Autodesk Fusion 360 part; units mm, degrees
note: some values were not read from the file. Chosen so that the rebuilt part matches the saved one: which bodies a step acts on. Set by a fixed rule: which sketch regions a step uses.
(part 4 of 5)
fillet "Fillet1'" radius 1 2 edges at (-68.425, -130.25, -19.5) (-53.825, -130.25, -19.5) on bodies 35 in component "edge-bracket_3d"
mirror "Mirror1" about plane through (0, 0, 0) normal (1, 0, 0) of bodies 35 makes body 36 in component "edge-bracket_3d"
pattern_circular "C-Pattern1''" count 4 over 360 about axis through (0, 0, 1.75) along (0, 0, 1) of bodies 35 36 makes body 37 at (139.5, -61.164856, -43.585564) makes body 38 at (61.164856, 139.5, -43.585564) makes body 39 at (-139.5, 61.164856, -43.585564) makes body 40 at (139.5, 61.164856, -43.585564) makes body 41 at (-61.164856, 139.5, -43.585564) makes body 42 at (-139.5, -61.164856, -43.585564) in component "edge-bracket_3d"
sketch "Sketch1 (4)" plane through (0, 139.5, 0) normal (0, 1, 0) x (-1, 0, 0) in component "sides"
  circle A0 centre (130.661165, -11.838835) radius 1.75
  circle A1 centre (130.661165, -37.161165) radius 1.75
  line L0 (122.236544, -3) -> (122.236544, -46)
  line L1 (122.236544, -46) -> (138.5, -46)
  line L2 (138.5, -46) -> (138.5, -3)
  line L3 (138.5, -3) -> (122.236544, -3)
  line L4 (142.5, -3) -> (-142.5, -3)
  line L5 (-142.5, -3) -> (-142.5, -46)
  line L6 (-142.5, -46) -> (142.5, -46)
  line L7 (142.5, -46) -> (142.5, -3)
  line L8 (139.5, -46) -> (139.5, -3)
  line L9 (142.5, -37.4) -> (139.5, -37.4)
  line L10 (142.5, -28.8) -> (139.5, -28.8)
  line L11 (142.5, -20.2) -> (139.5, -20.2)
  line L12 (142.5, -11.6) -> (139.5, -11.6)
  line L13 (142.5, -3) -> (139.5, -3)
  line L14 (0, -46) -> (0, -3) construction
  line L15 (-142.5, -37.4) -> (-139.5, -37.4)
  line L16 (-139.5, -46) -> (-139.5, -3)
  line L17 (-142.5, -28.8) -> (-139.5, -28.8)
  line L18 (-142.5, -20.2) -> (-139.5, -20.2)
  line L19 (-142.5, -11.6) -> (-139.5, -11.6)
  point P0 (143.5, -3)
  point P1 (139.5, -46)
  point P2 (-143.5, -3)
  point P3 (-139.5, -46)
  dimension "d354" = 3
  dimension "d355" = 3
  dimension "d356" = 8.6
  dimension "d357" = 43
  dimension "d360" = 0
  dimension "d361" = 34.4
  constraint horizontal L4
  constraint vertical L5
  constraint horizontal L6
  constraint vertical L7
  constraint coincident P3 L6
  constraint coincident P0 L4
  constraint coincident P1 L8.start
  constraint coincident L4 L8.end
  constraint perpendicular L4 L8
  constraint coincident L7 L9.start
  constraint coincident L8 L9.end
  constraint perpendicular L8 L9
  constraint midpoint L6 L14.start
  constraint midpoint L4 L14.end
  constraint symmetric P1 L14 P3
  constraint symmetric L8.end L14 L16.end
  constraint symmetric L9.start L14 L15.start
  constraint symmetric L9.end L14 L15.end
  constraint symmetric L10.start L14 L17.start
  constraint symmetric L10.end L14 L17.end
  constraint symmetric L11.start L14 L18.start
  constraint symmetric L11.end L14 L18.end
  constraint symmetric L12.start L14 L19.start
  constraint symmetric L12.end L14 L19.end
  measures "d354" distance of P1 L7
  measures "d355" distance of P3 L5
  measures "d356" distance of L6 L9
  measures "d357" distance of L4.start L6.end
extrude "Extrude1'''''" add sketch "Sketch1 (4)" along normal blind 3 separate body contours A0 | A1 | L0 L1 L2 L3 L4 L6 | L0 L4 L6 L16 | L2 L4 L6 L8 | L4 L7 L8 L12 L13 | L5 L16 L18 L19 | L6 L7 L8 L9 | L5 L15 L16 L17 | L7 L8 L10 L11 picked at (131.451099, -11.382766) picked at (129.871232, -36.705097) picked at (124.519186, -28.46729) picked at (34.991029, -23.066667) picked at (138.833333, -28.8) picked at (140.5, -8.733333) picked at (-141.5, -14.466667) picked at (140.5, -40.266667) picked at (-140.5, -34.533333) picked at (140.5, -23.066667) makes body 43 in component "sides"
sketch "Sketch2 (5)" plane through (0, 142.5, 0) normal (0, 1, 0) x (-1, 0, 0) in component "sides"
  line L0 (-142.5, -20.2) -> (-139.5, -20.2)
  line L1 (-139.5, -20.2) -> (-139.5, -28.8)
  line L2 (-139.5, -28.8) -> (-142.5, -28.8)
  line L3 (-142.5, -28.8) -> (-142.5, -37.4)
  line L4 (-142.5, -37.4) -> (-139.5, -37.4)
  line L5 (-139.5, -37.4) -> (-139.5, -46)
  line L6 (-139.5, -46) -> (142.5, -46)
  line L7 (142.5, -46) -> (142.5, -37.4)
  line L8 (142.5, -37.4) -> (139.5, -37.4)
  line L9 (139.5, -37.4) -> (139.5, -28.8)
  line L10 (139.5, -28.8) -> (142.5, -28.8)
  line L11 (142.5, -28.8) -> (142.5, -20.2)
  line L12 (142.5, -20.2) -> (139.5, -20.2)
  line L13 (139.5, -20.2) -> (139.5, -11.6)
  line L14 (139.5, -11.6) -> (142.5, -11.6)
  line L15 (142.5, -11.6) -> (142.5, -3)
  line L16 (142.5, -3) -> (-139.5, -3)
  line L17 (-139.5, -3) -> (-139.5, -11.6)
  line L18 (-139.5, -11.6) -> (-142.5, -11.6)
  line L19 (-142.5, -11.6) -> (-142.5, -20.2)
  circle A0 centre (130.661165, -11.838835) radius 1.75
  circle A1 centre (130.661165, -37.161165) radius 1.75
  line L20 (122.236544, -3) -> (122.236544, -46)
  line L21 (122.236544, -46) -> (138.5, -46)
  line L22 (138.5, -46) -> (138.5, -3)
  line L23 (138.5, -3) -> (122.236544, -3)
  line L24 (54.825, -3) -> (54.825, -46)
  line L25 (54.825, -46) -> (67.425, -46)
  line L26 (67.425, -46) -> (67.425, -3)
  line L27 (67.425, -3) -> (54.825, -3)
  circle A2 centre (61.125, -37.161165) radius 1.6
  circle A3 centre (61.125, -11.838835) radius 1.6
  line L28 (-54.825, -46) -> (-54.825, -3)
  line L29 (-54.825, -3) -> (-67.425, -3)
  line L30 (-67.425, -3) -> (-67.425, -46)
  line L31 (-67.425, -46) -> (-54.825, -46)
  circle A4 centre (-61.125, -37.161165) radius 1.6
  circle A5 centre (-61.125, -11.838835) radius 1.6
  circle A6 centre (-130.661165, -37.161165) radius 1.75
  circle A7 centre (-130.661165, -11.838835) radius 1.75
  line L32 (-122.236544, -46) -> (-122.236544, -3)
  line L33 (-122.236544, -3) -> (-138.5, -3)
  line L34 (-138.5, -3) -> (-138.5, -46)
  line L35 (-138.5, -46) -> (-122.236544, -46)
extrude "Extrude2'''" cut sketch "Sketch2 (5)" against normal blind 3 contours A0 | A1 | A2 | A3 | A4 | A5 | A6 | A7 picked at (131.451099, -11.382766) picked at (129.871232, -36.705097) picked at (61.391667, -36.38488) picked at (61.391667, -11.062549) picked at (-60.858333, -36.38488) picked at (-60.858333, -11.062549) picked at (-131.451099, -36.705097) picked at (-129.871232, -11.382766) bodies 43 in component "sides"
pattern_circular "C-Pattern1'''" count 4 over 360 about axis through (0, 0, 1.75) along (0, 0, 1) of bodies 43 makes body 44 at (-139.5, -19.873831, -28.537978) makes body 45 at (19.873831, -139.5, -28.537978) makes body 46 at (139.5, 19.873831, -28.537978) in component "sides"
sketch "Sketch3 (5)" plane through (0, 142.5, 0) normal (0, 1, 0) x (-1, 0, 0) in component "sides"
  circle A0 centre (-61.125, -11.838835) radius 1.6
  circle A1 centre (130.661165, -11.838835) radius 1.75
  circle A2 centre (61.125, -37.161165) radius 1.6
  circle A3 centre (-130.661165, -37.161165) radius 1.75
  circle A4 centre (-61.125, -37.161165) radius 1.6
  circle A5 centre (130.661165, -37.161165) radius 1.75
  circle A6 centre (61.125, -11.838835) radius 1.6
  circle A7 centre (-130.661165, -11.838835) radius 1.75
  line L0 (-142.5, -20.2) -> (-139.5, -20.2)
  line L1 (-139.5, -20.2) -> (-139.5, -28.8)
  line L2 (-139.5, -28.8) -> (-142.5, -28.8)
  line L3 (-142.5, -28.8) -> (-142.5, -37.4)
  line L4 (-142.5, -37.4) -> (-139.5, -37.4)
  line L5 (-139.5, -37.4) -> (-139.5, -46)
  line L6 (-139.5, -46) -> (142.5, -46)
  line L7 (142.5, -46) -> (142.5, -37.4)
  line L8 (142.5, -37.4) -> (139.5, -37.4)
  line L9 (139.5, -37.4) -> (139.5, -28.8)
  line L10 (139.5, -28.8) -> (142.5, -28.8)
  line L11 (142.5, -28.8) -> (142.5, -20.2)
  line L12 (142.5, -20.2) -> (139.5, -20.2)
  line L13 (139.5, -20.2) -> (139.5, -11.6)
  line L14 (139.5, -11.6) -> (142.5, -11.6)
  line L15 (142.5, -11.6) -> (142.5, -3)
  line L16 (142.5, -3) -> (-139.5, -3)
  line L17 (-139.5, -3) -> (-139.5, -11.6)
  line L18 (-139.5, -11.6) -> (-142.5, -11.6)
  line L19 (-142.5, -11.6) -> (-142.5, -20.2)
  line L20 (61.125, -37.161165) -> (-61.125, -11.838835) construction
  line L21 (0, -24.5) -> (0, -46) construction
  line L22 (122.25, -21) -> (-122.25, -21)
  circle A8 centre (0, -33.5) radius 5.5
  dimension "d368" = 11
  dimension "d369" = 25
  dimension "d370" = 12.5
  constraint midpoint L20 L21.start
  constraint coincident L6 L21.end
  constraint perpendicular L6 L21
  constraint coincident L21 A8.centre
  measures "d368" diameter of A8
  measures "d369" distance of L6 L22
  measures "d370" distance of L22 A8.centre
extrude "Extrude3''''" cut sketch "Sketch3 (5)" against normal blind 282 contours A8 picked at (0.137005, -35.084997) bodies 43 in component "sides"
sketch "Sketch3 (6)" plane through (0, 0, -18) normal (0, 0, -1) x (1, 0, 0) in component "bolt-holder_3d"
  arc A0 (-68.625, 128.75) -> (-69.625, 129.75) centre (-69.625, 128.75) ccw
  line L0 (-69.625, 129.75) -> (-116.02505, 129.75)
  arc A1 (-116.02505, 129.75) -> (-116.716711, 128.027778) centre (-116.02505, 128.75) ccw
  arc A2 (-115.999634, 117.256712) -> (-116.716711, 128.027778) centre (-122.25, 122.25) ccw
  arc A3 (-115.999634, 117.256712) -> (-115.925445, 115.925445) centre (-115.218338, 116.632551) ccw
  line L1 (-115.925445, 115.925445) -> (-101.292893, 101.292893)
  arc A4 (-101.292893, 101.292893) -> (-100.585786, 101) centre (-100.585786, 102) ccw
  line L2 (-100.585786, 101) -> (-99.5, 101)
  line L3 (-99.5, 101) -> (-99.5, 110.5)
  line L4 (-99.5, 110.5) -> (-87.5, 110.5)
  line L5 (-87.5, 110.5) -> (-87.5, 101)
  line L6 (-87.5, 101) -> (-87, 101)
  arc A5 (-87, 101) -> (-86, 102) centre (-87, 102) ccw
  line L7 (-86, 102) -> (-86, 108.5)
  line L8 (-86, 108.5) -> (-84, 108.5)
  line L9 (-84, 108.5) -> (-84, 102)
  arc A6 (-84, 102) -> (-83, 101) centre (-83, 102) ccw
  line L10 (-83, 101) -> (-82.5, 101)
  line L11 (-82.5, 101) -> (-82.5, 110.5)
  line L12 (-82.5, 110.5) -> (-70.5, 110.5)
  line L13 (-70.5, 110.5) -> (-70.5, 101)
  line L14 (-70.5, 101) -> (-70, 101)
  arc A7 (-70, 101) -> (-69, 102) centre (-70, 102) ccw
  line L15 (-69, 102) -> (-69, 108.5)
  line L16 (-69, 108.5) -> (-67, 108.5)
  line L17 (-67, 108.5) -> (-67, 102)
  arc A8 (-67, 102) -> (-66, 101) centre (-66, 102) ccw
  line L18 (-66, 101) -> (-65.5, 101)
  line L19 (-65.5, 101) -> (-65.5, 110.5)
  line L20 (-65.5, 110.5) -> (-53.5, 110.5)
  line L21 (-53.5, 110.5) -> (-53.5, 101)
  line L22 (-53.5, 101) -> (-53, 101)
  arc A9 (-53, 101) -> (-52, 102) centre (-53, 102) ccw
  line L23 (-52, 102) -> (-52, 108.5)
  line L24 (-52, 108.5) -> (-50, 108.5)
  line L25 (-50, 108.5) -> (-50, 102)
  arc A10 (-50, 102) -> (-49, 101) centre (-49, 102) ccw
  line L26 (-49, 101) -> (-48.5, 101)
  line L27 (-48.5, 101) -> (-48.5, 110.5)
  line L28 (-48.5, 110.5) -> (-36.5, 110.5)
  line L29 (-36.5, 110.5) -> (-36.5, 101)
  line L30 (-36.5, 101) -> (-36, 101)
  arc A11 (-36, 101) -> (-35, 102) centre (-36, 102) ccw
  line L31 (-35, 102) -> (-35, 108.5)
  line L32 (-35, 108.5) -> (-33, 108.5)
  line L33 (-33, 108.5) -> (-33, 102)
  arc A12 (-33, 102) -> (-32, 101) centre (-32, 102) ccw
  line L34 (-32, 101) -> (-31.5, 101)
  line L35 (-31.5, 101) -> (-31.5, 110.5)
  line L36 (-31.5, 110.5) -> (-19.5, 110.5)
  line L37 (-19.5, 110.5) -> (-19.5, 101)
  line L38 (-19.5, 101) -> (-19, 101)
  arc A13 (-19, 101) -> (-18, 102) centre (-19, 102) ccw
  line L39 (-18, 102) -> (-18, 108.5)
  line L40 (-18, 108.5) -> (-16, 108.5)
  line L41 (-16, 108.5) -> (-16, 102)
  arc A14 (-16, 102) -> (-15, 101) centre (-15, 102) ccw
  line L42 (-15, 101) -> (-14.5, 101)
  line L43 (-14.5, 101) -> (-14.5, 110.5)
  line L44 (-14.5, 110.5) -> (-2.5, 110.5)
  line L45 (-2.5, 110.5) -> (-2.5, 101)
  line L46 (-2.5, 101) -> (-2, 101)
  arc A15 (-2, 101) -> (-1, 102) centre (-2, 102) ccw
  line L47 (-1, 102) -> (-1, 108.5)
  line L48 (-1, 108.5) -> (1, 108.5)
  line L49 (1, 108.5) -> (1, 102)
  arc A16 (1, 102) -> (2, 101) centre (2, 102) ccw
  line L50 (2, 101) -> (2.5, 101)
  line L51 (2.5, 101) -> (2.5, 110.5)
  line L52 (2.5, 110.5) -> (14.5, 110.5)
  line L53 (14.5, 110.5) -> (14.5, 101)
  line L54 (14.5, 101) -> (15, 101)
  arc A17 (15, 101) -> (16, 102) centre (15, 102) ccw
  line L55 (16, 102) -> (16, 108.5)
  line L56 (16, 108.5) -> (18, 108.5)
  line L57 (18, 108.5) -> (18, 102)
  arc A18 (18, 102) -> (19, 101) centre (19, 102) ccw
  line L58 (19, 101) -> (19.5, 101)
  line L59 (19.5, 101) -> (19.5, 110.5)
  line L60 (19.5, 110.5) -> (31.5, 110.5)
  line L61 (31.5, 110.5) -> (31.5, 101)
  line L62 (31.5, 101) -> (32, 101)
  arc A19 (32, 101) -> (33, 102) centre (32, 102) ccw
  line L63 (33, 102) -> (33, 108.5)
  line L64 (33, 108.5) -> (35, 108.5)
  line L65 (35, 108.5) -> (35, 102)
  arc A20 (35, 102) -> (36, 101) centre (36, 102) ccw
  line L66 (36, 101) -> (36.5, 101)
  line L67 (36.5, 101) -> (36.5, 110.5)
  line L68 (36.5, 110.5) -> (48.5, 110.5)
  line L69 (48.5, 110.5) -> (48.5, 101)
  line L70 (48.5, 101) -> (49, 101)
  arc A21 (49, 101) -> (50, 102) centre (49, 102) ccw
  line L71 (50, 102) -> (50, 108.5)
  line L72 (50, 108.5) -> (52, 108.5)
  line L73 (52, 108.5) -> (52, 102)
  arc A22 (52, 102) -> (53, 101) centre (53, 102) ccw
  line L74 (53, 101) -> (53.5, 101)
  line L75 (53.5, 101) -> (53.5, 110.5)
  line L76 (53.5, 110.5) -> (65.5, 110.5)
  line L77 (65.5, 110.5) -> (65.5, 101)
  line L78 (65.5, 101) -> (66, 101)
  arc A23 (66, 101) -> (67, 102) centre (66, 102) ccw
  line L79 (67, 102) -> (67, 108.5)
  line L80 (67, 108.5) -> (69, 108.5)
  line L81 (69, 108.5) -> (69, 102)
  arc A24 (69, 102) -> (70, 101) centre (70, 102) ccw
  line L82 (70, 101) -> (70.5, 101)
  line L83 (70.5, 101) -> (70.5, 110.5)
  line L84 (70.5, 110.5) -> (82.5, 110.5)
  line L85 (82.5, 110.5) -> (82.5, 101)
  line L86 (82.5, 101) -> (83, 101)
  arc A25 (83, 101) -> (84, 102) centre (83, 102) ccw
  line L87 (84, 102) -> (84, 108.5)
  line L88 (84, 108.5) -> (86, 108.5)
  line L89 (86, 108.5) -> (86, 102)
  arc A26 (86, 102) -> (87, 101) centre (87, 102) ccw
  line L90 (87, 101) -> (87.5, 101)
  line L91 (87.5, 101) -> (87.5, 110.5)
  line L92 (87.5, 110.5) -> (99.5, 110.5)
  line L93 (99.5, 110.5) -> (99.5, 101)
  line L94 (99.5, 101) -> (100.585786, 101)
  arc A27 (100.585786, 101) -> (101.292893, 101.292893) centre (100.585786, 102) ccw
  line L95 (101.292893, 101.292893) -> (116.946699, 116.946699)
  arc A28 (116.946699, 116.946699) -> (122.25, 129.75) centre (122.25, 122.25) ccw
  line L96 (122.25, 129.75) -> (69.625, 129.75)
  arc A29 (69.625, 129.75) -> (68.625, 128.75) centre (69.625, 128.75) ccw
  line L97 (68.625, 128.75) -> (68.625, 122.25)
  arc A30 (53.625, 122.25) -> (68.625, 122.25) centre (61.125, 122.25) ccw
  line L98 (53.625, 122.25) -> (53.625, 128.75)
  arc A31 (53.625, 128.75) -> (52.625, 129.75) centre (52.625, 128.75) ccw
  line L99 (52.625, 129.75) -> (-52.625, 129.75)
  arc A32 (-52.625, 129.75) -> (-53.625, 128.75) centre (-52.625, 128.75) ccw
  line L100 (-53.625, 128.75) -> (-53.625, 122.25)
  arc A33 (-68.625, 122.25) -> (-53.625, 122.25) centre (-61.125, 122.25) ccw
  line L101 (-68.625, 122.25) -> (-68.625, 128.75)
  circle A34 centre (122.25, 122.25) radius 2.5
  line L102 (-12.5, 124.5) -> (-4.5, 124.5)
  arc A35 (4.5, 124.5) -> (-4.5, 124.5) centre (0, 118.5) ccw
  line L103 (4.5, 124.5) -> (12.5, 124.5)
  arc A36 (21.5, 124.5) -> (12.5, 124.5) centre (17, 118.5) ccw
  line L104 (21.5, 124.5) -> (29.5, 124.5)
  arc A37 (38.5, 124.5) -> (29.5, 124.5) centre (34, 118.5) ccw
  line L105 (38.5, 124.5) -> (51, 124.5)
  line L106 (51, 124.5) -> (51, 112.5)
  line L107 (51, 112.5) -> (38.5, 112.5)
  arc A38 (29.5, 112.5) -> (38.5, 112.5) centre (34, 118.5) ccw
  line L108 (29.5, 112.5) -> (21.5, 112.5)
  arc A39 (12.5, 112.5) -> (21.5, 112.5) centre (17, 118.5) ccw
  line L109 (12.5, 112.5) -> (4.5, 112.5)
  arc A40 (-4.5, 112.5) -> (4.5, 112.5) centre (0, 118.5) ccw
  line L110 (-4.5, 112.5) -> (-12.5, 112.5)
  arc A41 (-21.5, 112.5) -> (-12.5, 112.5) centre (-17, 118.5) ccw
  line L111 (-21.5, 112.5) -> (-29.5, 112.5)
  arc A42 (-38.5, 112.5) -> (-29.5, 112.5) centre (-34, 118.5) ccw
  line L112 (-38.5, 112.5) -> (-51, 112.5)
  line L113 (-51, 112.5) -> (-51, 124.5)
  line L114 (-51, 124.5) -> (-38.5, 124.5)
  arc A43 (-29.5, 124.5) -> (-38.5, 124.5) centre (-34, 118.5) ccw
  line L115 (-29.5, 124.5) -> (-21.5, 124.5)
  arc A44 (-12.5, 124.5) -> (-21.5, 124.5) centre (-17, 118.5) ccw
  arc A45 (-29.5, 112.5) -> (-29.5, 124.5) centre (-34, 118.5) ccw
  line L116 (-29.5, 112.5) -> (-21.5, 112.5)
  arc A46 (-21.5, 124.5) -> (-21.5, 112.5) centre (-17, 118.5) ccw
  line L117 (-21.5, 124.5) -> (-29.5, 124.5)
  line L118 (-51, 124.5) -> (-51, 112.5)
  line L119 (-51, 112.5) -> (-38.5, 112.5)
  arc A47 (-38.5, 124.5) -> (-38.5, 112.5) centre (-34, 118.5) ccw
  line L120 (-38.5, 124.5) -> (-51, 124.5)
  arc A48 (-12.5, 112.5) -> (-12.5, 124.5) centre (-17, 118.5) ccw
  line L121 (-12.5, 112.5) -> (-4.5, 112.5)
  arc A49 (-4.5, 124.5) -> (-4.5, 112.5) centre (0, 118.5) ccw
  line L122 (-4.5, 124.5) -> (-12.5, 124.5)
  arc A50 (4.5, 112.5) -> (4.5, 124.5) centre (0, 118.5) ccw
  line L123 (4.5, 112.5) -> (12.5, 112.5)
  arc A51 (12.5, 124.5) -> (12.5, 112.5) centre (17, 118.5) ccw
  line L124 (12.5, 124.5) -> (4.5, 124.5)
  arc A52 (21.5, 112.5) -> (21.5, 124.5) centre (17, 118.5) ccw
  line L125 (21.5, 112.5) -> (29.5, 112.5)
  arc A53 (29.5, 124.5) -> (29.5, 112.5) centre (34, 118.5) ccw
  line L126 (29.5, 124.5) -> (21.5, 124.5)
  line L127 (51, 124.5) -> (38.5, 124.5)
  arc A54 (38.5, 112.5) -> (38.5, 124.5) centre (34, 118.5) ccw
  line L128 (38.5, 112.5) -> (51, 112.5)
  line L129 (51, 112.5) -> (51, 124.5)
  line L130 (110.5, 70.5) -> (105.75, 70.5)
  line L131 (105.75, 70.5) -> (105.75, 82.5)
  line L132 (105.75, 82.5) -> (110.5, 82.5)
  line L133 (110.5, 82.5) -> (110.5, 70.5)
  circle A55 centre (122.25, 61.125) radius 1.6
  line L134 (110.5, 87.5) -> (105.75, 87.5)
  line L135 (105.75, 87.5) -> (105.75, 99.5)
  line L136 (105.75, 99.5) -> (110.5, 99.5)
  line L137 (110.5, 99.5) -> (110.5, 87.5)
  line L138 (51, -124.5) -> (46.25, -124.5)
  line L139 (46.25, -124.5) -> (46.25, -112.5)
  line L140 (46.25, -112.5) -> (51, -112.5)
  line L141 (51, -112.5) -> (51, -124.5)
  circle A56 centre (0, 118.5) radius 7.5
  circle A57 centre (-61.125, -122.25) radius 1.6
  circle A58 centre (61.125, -122.25) radius 1.6
  circle A59 centre (122.25, -61.125) radius 1.6
  circle A60 centre (-61.125, 122.25) radius 1.6
  circle A61 centre (61.125, 122.25) radius 1.6
  circle A62 centre (-122.25, -61.125) radius 1.6
  circle A63 centre (-122.25, 61.125) radius 1.6
  circle A64 centre (-34, 123) radius 1.6
  circle A65 centre (-17, 123) radius 1.6
  circle A66 centre (17, 123) radius 1.6
  circle A67 centre (34, 123) radius 1.6
  circle A68 centre (-34, 114) radius 1.6
  circle A69 centre (17, 114) radius 1.6
  circle A70 centre (-17, 114) radius 1.6
  circle A71 centre (34, 114) radius 1.6
  circle A72 centre (-122.25, 122.25) radius 2.5
  circle A73 centre (-122.25, -122.25) radius 2.5
  line L142 (-105.75, -2.5) -> (-105.75, -14.5)
  line L143 (-105.75, -14.5) -> (-110.5, -14.5)
  line L144 (-110.5, -14.5) -> (-110.5, -2.5)
  line L145 (-110.5, -2.5) -> (-105.75, -2.5)
  line L146 (-105.75, -87.5) -> (-105.75, -99.5)
  line L147 (-105.75, -99.5) -> (-110.5, -99.5)
  line L148 (-110.5, -99.5) -> (-110.5, -87.5)
  line L149 (-110.5, -87.5) -> (-105.75, -87.5)
  circle A74 centre (122.25, 122.25) radius 2.5
  line L150 (-105.75, -19.5) -> (-105.75, -31.5)
  line L151 (-105.75, -31.5) -> (-110.5, -31.5)
  line L152 (-110.5, -31.5) -> (-110.5, -19.5)
  line L153 (-110.5, -19.5) -> (-105.75, -19.5)
  line L154 (-105.75, -36.5) -> (-105.75, -48.5)
  line L155 (-105.75, -48.5) -> (-110.5, -48.5)
  line L156 (-110.5, -48.5) -> (-110.5, -36.5)
  line L157 (-110.5, -36.5) -> (-105.75, -36.5)
  line L158 (-105.75, -53.5) -> (-105.75, -65.5)
  line L159 (-105.75, -65.5) -> (-110.5, -65.5)
  line L160 (-110.5, -65.5) -> (-110.5, -53.5)
  line L161 (-110.5, -53.5) -> (-105.75, -53.5)
  line L162 (-105.75, -70.5) -> (-105.75, -82.5)
  line L163 (-105.75, -82.5) -> (-110.5, -82.5)
  line L164 (-110.5, -82.5) -> (-110.5, -70.5)
  line L165 (-110.5, -70.5) -> (-105.75, -70.5)
  line L166 (-46.25, -112.5) -> (-46.25, -124.5)
  line L167 (-46.25, -124.5) -> (-51, -124.5)
  line L168 (-51, -124.5) -> (-51, -112.5)
  line L169 (-51, -112.5) -> (-46.25, -112.5)
  line L170 (-105.75, 14.5) -> (-105.75, 2.5)
  line L171 (-105.75, 2.5) -> (-110.5, 2.5)
  line L172 (-110.5, 2.5) -> (-110.5, 14.5)
  line L173 (-110.5, 14.5) -> (-105.75, 14.5)
  line L174 (-105.75, 31.5) -> (-105.75, 19.5)
  line L175 (-105.75, 19.5) -> (-110.5, 19.5)
  line L176 (-110.5, 19.5) -> (-110.5, 31.5)
  line L177 (-110.5, 31.5) -> (-105.75, 31.5)
  line L178 (-105.75, 48.5) -> (-105.75, 36.5)
  line L179 (-105.75, 36.5) -> (-110.5, 36.5)
  line L180 (-110.5, 36.5) -> (-110.5, 48.5)
  line L181 (-110.5, 48.5) -> (-105.75, 48.5)
  line L182 (-105.75, 65.5) -> (-105.75, 53.5)
  line L183 (-105.75, 53.5) -> (-110.5, 53.5)
  line L184 (-110.5, 53.5) -> (-110.5, 65.5)
  line L185 (-110.5, 65.5) -> (-105.75, 65.5)
  line L186 (-105.75, 82.5) -> (-105.75, 70.5)
  line L187 (-105.75, 70.5) -> (-110.5, 70.5)
  line L188 (-110.5, 70.5) -> (-110.5, 82.5)
  line L189 (-110.5, 82.5) -> (-105.75, 82.5)
  line L190 (-105.75, 99.5) -> (-105.75, 87.5)
  line L191 (-105.75, 87.5) -> (-110.5, 87.5)
  line L192 (-110.5, 87.5) -> (-110.5, 99.5)
  line L193 (-110.5, 99.5) -> (-105.75, 99.5)
  line L194 (110.5, -99.5) -> (105.75, -99.5)
  line L195 (105.75, -99.5) -> (105.75, -87.5)
  line L196 (105.75, -87.5) -> (110.5, -87.5)
  line L197 (110.5, -87.5) -> (110.5, -99.5)
  line L198 (110.5, -82.5) -> (105.75, -82.5)
  line L199 (105.75, -82.5) -> (105.75, -70.5)
  line L200 (105.75, -70.5) -> (110.5, -70.5)
  line L201 (110.5, -70.5) -> (110.5, -82.5)
  line L202 (110.5, -65.5) -> (105.75, -65.5)
  line L203 (105.75, -65.5) -> (105.75, -53.5)
  line L204 (105.75, -53.5) -> (110.5, -53.5)
  line L205 (110.5, -53.5) -> (110.5, -65.5)
  line L206 (110.5, -48.5) -> (105.75, -48.5)
  line L207 (105.75, -48.5) -> (105.75, -36.5)
  line L208 (105.75, -36.5) -> (110.5, -36.5)
  line L209 (110.5, -36.5) -> (110.5, -48.5)
  line L210 (110.5, -31.5) -> (105.75, -31.5)
  line L211 (105.75, -31.5) -> (105.75, -19.5)
  line L212 (105.75, -19.5) -> (110.5, -19.5)
  line L213 (110.5, -19.5) -> (110.5, -31.5)
  line L214 (110.5, 36.5) -> (105.75, 36.5)
  line L215 (105.75, 36.5) -> (105.75, 48.5)
  line L216 (105.75, 48.5) -> (110.5, 48.5)
  line L217 (110.5, 48.5) -> (110.5, 36.5)
  line L218 (110.5, -14.5) -> (105.75, -14.5)
  line L219 (105.75, -14.5) -> (105.75, -2.5)
  line L220 (105.75, -2.5) -> (110.5, -2.5)
  line L221 (110.5, -2.5) -> (110.5, -14.5)
  line L222 (110.5, 53.5) -> (105.75, 53.5)
  line L223 (105.75, 53.5) -> (105.75, 65.5)
  line L224 (105.75, 65.5) -> (110.5, 65.5)
  line L225 (110.5, 65.5) -> (110.5, 53.5)
  line L226 (110.5, 2.5) -> (105.75, 2.5)
  line L227 (105.75, 2.5) -> (105.75, 14.5)
  line L228 (105.75, 14.5) -> (110.5, 14.5)
  line L229 (110.5, 14.5) -> (110.5, 2.5)
  line L230 (110.5, 19.5) -> (105.75, 19.5)
  line L231 (105.75, 19.5) -> (105.75, 31.5)
  line L232 (105.75, 31.5) -> (110.5, 31.5)
  line L233 (110.5, 31.5) -> (110.5, 19.5)
  circle A75 centre (122.25, -122.25) radius 2.5
  arc A76 (-129.75, -122.25) -> (-122.25, -129.75) centre (-122.25, -122.25) ccw
  line L234 (-122.25, -129.75) -> (122.25, -129.75)
  arc A77 (122.25, -129.75) -> (129.75, -122.25) centre (122.25, -122.25) ccw
  line L235 (129.75, -122.25) -> (129.75, 122.25)
  arc A78 (129.75, 122.25) -> (122.25, 129.75) centre (122.25, 122.25) ccw
  line L236 (122.25, 129.75) -> (-122.25, 129.75)
  arc A79 (-122.25, 129.75) -> (-129.75, 122.25) centre (-122.25, 122.25) ccw
  line L237 (-129.75, 122.25) -> (-129.75, -122.25)
  line L238 (-35.732051, 126) -> (-37.464102, 123)
  line L239 (-37.464102, 123) -> (-35.732051, 120)
  line L240 (-35.732051, 120) -> (-32.267949, 120)
  line L241 (-32.267949, 120) -> (-30.535898, 123)
  line L242 (-30.535898, 123) -> (-32.267949, 126)
  line L243 (-32.267949, 126) -> (-35.732051, 126)
  line L244 (-34, 118.5) -> (-17, 118.5) construction
  line L245 (-8.5, 124.5) -> (-8.5, 112.5)
  line L246 (-25.5, 124.5) -> (-25.5, 112.5) construction
  line L247 (-42.5, 124.5) -> (-42.5, 112.5)
  line L248 (-35.732051, 117) -> (-32.267949, 117)
  line L249 (-32.267949, 117) -> (-30.535898, 114)
  line L250 (-30.535898, 114) -> (-32.267949, 111)
  line L251 (-32.267949, 111) -> (-35.732051, 111)
  line L252 (-35.732051, 111) -> (-37.464102, 114)
  line L253 (-37.464102, 114) -> (-35.732051, 117)
  line L254 (-15.267949, 126) -> (-13.535898, 123)
  line L255 (-13.535898, 123) -> (-15.267949, 120)
  line L256 (-15.267949, 120) -> (-18.732051, 120)
  line L257 (-18.732051, 120) -> (-20.464102, 123)
  line L258 (-20.464102, 123) -> (-18.732051, 126)
  line L259 (-18.732051, 126) -> (-15.267949, 126)
  line L260 (-15.267949, 117) -> (-18.732051, 117)
  line L261 (-13.535898, 114) -> (-15.267949, 117)
  line L262 (-15.267949, 111) -> (-13.535898, 114)
  line L263 (-18.732051, 111) -> (-15.267949, 111)
  line L264 (-20.464102, 114) -> (-18.732051, 111)
  line L265 (-18.732051, 117) -> (-20.464102, 114)
  point P0 (-34, 123)
  dimension "d392" = 3
  constraint coincident P0 A64.centre
  constraint horizontal L240
  constraint coincident A42.centre A43.centre
  constraint coincident A41.centre A44.centre
  constraint midpoint L102 L245.start
  constraint midpoint L121 L245.end
  constraint midpoint L115 L246.start
  constraint midpoint L111 L246.end
  constraint symmetric L245.start L246 L247.start
  constraint symmetric L245.end L246 L247.end
  measures "d392" distance of P0 L243
extrude "Extrude2''''" add sketch "Sketch3 (6)" against normal blind 2.5 separate body contours A41 A44 A46 A48 L254 L255 L256 L257 L258 L260 L261 L262 L264 L265 | L102 L110 A48 L121 L122 L245 | L111 L115 A45 L116 A46 L117 | A42 A43 A45 A47 L238 L239 L240 L241 L242 L248 L249 L250 L252 L253 | L112 L114 L119 A47 L120 L247 picked at (-13.351657, 118.678175) picked at (-8.839691, 118.678175) picked at (-25.009344, 115.233041) picked at (-37.648343, 118.678175) picked at (-42.160309, 118.321825) makes body 47 in component "bolt-holder_3d"
sketch "Sketch4 (3)" plane through (0, 0, -15.5) normal (0, 0, 1) x (-1, 0, 0) in component "bolt-holder_3d"
  arc A0 (12.5, 112.5) -> (15.131402, 111.236506) centre (17, 118.5) ccw
  line L0 (15.131402, 111.236506) -> (13.535898, 114)
  line L1 (13.535898, 114) -> (15.267949, 117)
  line L2 (15.267949, 117) -> (18.732051, 117)
  line L3 (18.732051, 117) -> (20.464102, 114)
  line L4 (20.464102, 114) -> (18.868598, 111.236506)
  arc A1 (18.868598, 111.236506) -> (21.5, 112.5) centre (17, 118.5) ccw
  line L5 (21.5, 112.5) -> (29.5, 112.5)
  arc A2 (29.5, 112.5) -> (32.131402, 111.236506) centre (34, 118.5) ccw
  line L6 (32.131402, 111.236506) -> (30.535898, 114)
  line L7 (30.535898, 114) -> (32.267949, 117)
  line L8 (32.267949, 117) -> (35.732051, 117)
  line L9 (35.732051, 117) -> (37.464102, 114)
  line L10 (37.464102, 114) -> (35.868598, 111.236506)
  arc A3 (35.868598, 111.236506) -> (38.5, 112.5) centre (34, 118.5) ccw
  line L11 (38.5, 112.5) -> (42.5, 112.5)
  line L12 (42.5, 112.5) -> (42.5, 124.5)
  line L13 (42.5, 124.5) -> (38.5, 124.5)
  arc A4 (38.5, 124.5) -> (35.868598, 125.763494) centre (34, 118.5) ccw
  line L14 (35.868598, 125.763494) -> (37.464102, 123)
  line L15 (37.464102, 123) -> (35.732051, 120)
  line L16 (35.732051, 120) -> (32.267949, 120)
  line L17 (32.267949, 120) -> (30.535898, 123)
  line L18 (30.535898, 123) -> (32.131402, 125.763494)
  arc A5 (32.131402, 125.763494) -> (29.5, 124.5) centre (34, 118.5) ccw
  line L19 (29.5, 124.5) -> (21.5, 124.5)
  arc A6 (21.5, 124.5) -> (18.868598, 125.763494) centre (17, 118.5) ccw
  line L20 (18.868598, 125.763494) -> (20.464102, 123)
  line L21 (20.464102, 123) -> (18.732051, 120)
  line L22 (18.732051, 120) -> (15.267949, 120)
  line L23 (15.267949, 120) -> (13.535898, 123)
  line L24 (13.535898, 123) -> (15.131402, 125.763494)
  arc A7 (15.131402, 125.763494) -> (12.5, 124.5) centre (17, 118.5) ccw
  line L25 (12.5, 124.5) -> (8.5, 124.5)
  line L26 (8.5, 124.5) -> (8.5, 112.5)
  line L27 (8.5, 112.5) -> (12.5, 112.5)
  line L28 (-110.5, 70.5) -> (-105.75, 70.5)
  line L29 (-105.75, 70.5) -> (-105.75, 82.5)
  line L30 (-105.75, 82.5) -> (-110.5, 82.5)
  line L31 (-110.5, 82.5) -> (-110.5, 70.5)
  circle A8 centre (-122.25, 61.125) radius 1.6
  line L32 (-110.5, 87.5) -> (-105.75, 87.5)
  line L33 (-105.75, 87.5) -> (-105.75, 99.5)
  line L34 (-105.75, 99.5) -> (-110.5, 99.5)
  line L35 (-110.5, 99.5) -> (-110.5, 87.5)
  line L36 (-51, -124.5) -> (-46.25, -124.5)
  line L37 (-46.25, -124.5) -> (-46.25, -112.5)
  line L38 (-46.25, -112.5) -> (-51, -112.5)
  line L39 (-51, -112.5) -> (-51, -124.5)
  circle A9 centre (0, 118.5) radius 7.5
  circle A10 centre (61.125, -122.25) radius 1.6
  circle A11 centre (-61.125, -122.25) radius 1.6
  circle A12 centre (-122.25, -61.125) radius 1.6
  circle A13 centre (61.125, 122.25) radius 1.6
  circle A14 centre (-61.125, 122.25) radius 1.6
  circle A15 centre (122.25, -61.125) radius 1.6
  circle A16 centre (122.25, 61.125) radius 1.6
  circle A17 centre (34, 123) radius 1.6
  circle A18 centre (17, 123) radius 1.6
  circle A19 centre (-17, 123) radius 1.6
  circle A20 centre (-34, 123) radius 1.6
  circle A21 centre (34, 114) radius 1.6
  circle A22 centre (-17, 114) radius 1.6
  circle A23 centre (17, 114) radius 1.6
  circle A24 centre (-34, 114) radius 1.6
  circle A25 centre (122.25, 122.25) radius 2.5
  circle A26 centre (122.25, -122.25) radius 2.5
  line L40 (105.75, -2.5) -> (105.75, -14.5)
  line L41 (105.75, -14.5) -> (110.5, -14.5)
  line L42 (110.5, -14.5) -> (110.5, -2.5)
  line L43 (110.5, -2.5) -> (105.75, -2.5)
  line L44 (105.75, -87.5) -> (105.75, -99.5)
  line L45 (105.75, -99.5) -> (110.5, -99.5)
  line L46 (110.5, -99.5) -> (110.5, -87.5)
  line L47 (110.5, -87.5) -> (105.75, -87.5)
  circle A27 centre (-122.25, 122.25) radius 2.5
  line L48 (105.75, -19.5) -> (105.75, -31.5)
  line L49 (105.75, -31.5) -> (110.5, -31.5)
  line L50 (110.5, -31.5) -> (110.5, -19.5)
  line L51 (110.5, -19.5) -> (105.75, -19.5)
  line L52 (105.75, -36.5) -> (105.75, -48.5)
  line L53 (105.75, -48.5) -> (110.5, -48.5)
  line L54 (110.5, -48.5) -> (110.5, -36.5)
  line L55 (110.5, -36.5) -> (105.75, -36.5)
  line L56 (105.75, -53.5) -> (105.75, -65.5)
  line L57 (105.75, -65.5) -> (110.5, -65.5)
  line L58 (110.5, -65.5) -> (110.5, -53.5)
  line L59 (110.5, -53.5) -> (105.75, -53.5)
  line L60 (105.75, -70.5) -> (105.75, -82.5)
  line L61 (105.75, -82.5) -> (110.5, -82.5)
  line L62 (110.5, -82.5) -> (110.5, -70.5)
  line L63 (110.5, -70.5) -> (105.75, -70.5)
  line L64 (46.25, -112.5) -> (46.25, -124.5)
  line L65 (46.25, -124.5) -> (51, -124.5)
  line L66 (51, -124.5) -> (51, -112.5)
  line L67 (51, -112.5) -> (46.25, -112.5)
  line L68 (105.75, 14.5) -> (105.75, 2.5)
  line L69 (105.75, 2.5) -> (110.5, 2.5)
  line L70 (110.5, 2.5) -> (110.5, 14.5)
  line L71 (110.5, 14.5) -> (105.75, 14.5)
  line L72 (105.75, 31.5) -> (105.75, 19.5)
  line L73 (105.75, 19.5) -> (110.5, 19.5)
  line L74 (110.5, 19.5) -> (110.5, 31.5)
  line L75 (110.5, 31.5) -> (105.75, 31.5)
  line L76 (105.75, 48.5) -> (105.75, 36.5)
  line L77 (105.75, 36.5) -> (110.5, 36.5)
  line L78 (110.5, 36.5) -> (110.5, 48.5)
  line L79 (110.5, 48.5) -> (105.75, 48.5)
  line L80 (105.75, 65.5) -> (105.75, 53.5)
  line L81 (105.75, 53.5) -> (110.5, 53.5)
  line L82 (110.5, 53.5) -> (110.5, 65.5)
  line L83 (110.5, 65.5) -> (105.75, 65.5)
  line L84 (105.75, 82.5) -> (105.75, 70.5)
  line L85 (105.75, 70.5) -> (110.5, 70.5)
  line L86 (110.5, 70.5) -> (110.5, 82.5)
  line L87 (110.5, 82.5) -> (105.75, 82.5)
  line L88 (105.75, 99.5) -> (105.75, 87.5)
  line L89 (105.75, 87.5) -> (110.5, 87.5)
  line L90 (110.5, 87.5) -> (110.5, 99.5)
  line L91 (110.5, 99.5) -> (105.75, 99.5)
  line L92 (-110.5, -99.5) -> (-105.75, -99.5)
  line L93 (-105.75, -99.5) -> (-105.75, -87.5)
  line L94 (-105.75, -87.5) -> (-110.5, -87.5)
  line L95 (-110.5, -87.5) -> (-110.5, -99.5)
  line L96 (-110.5, -82.5) -> (-105.75, -82.5)
  line L97 (-105.75, -82.5) -> (-105.75, -70.5)
  line L98 (-105.75, -70.5) -> (-110.5, -70.5)
  line L99 (-110.5, -70.5) -> (-110.5, -82.5)
  line L100 (-110.5, -65.5) -> (-105.75, -65.5)
  line L101 (-105.75, -65.5) -> (-105.75, -53.5)
  line L102 (-105.75, -53.5) -> (-110.5, -53.5)
  line L103 (-110.5, -53.5) -> (-110.5, -65.5)
  line L104 (-110.5, -48.5) -> (-105.75, -48.5)
  line L105 (-105.75, -48.5) -> (-105.75, -36.5)
  line L106 (-105.75, -36.5) -> (-110.5, -36.5)
  line L107 (-110.5, -36.5) -> (-110.5, -48.5)
  line L108 (-110.5, -31.5) -> (-105.75, -31.5)
  line L109 (-105.75, -31.5) -> (-105.75, -19.5)
  line L110 (-105.75, -19.5) -> (-110.5, -19.5)
  line L111 (-110.5, -19.5) -> (-110.5, -31.5)
  line L112 (-110.5, 36.5) -> (-105.75, 36.5)
  line L113 (-105.75, 36.5) -> (-105.75, 48.5)
  line L114 (-105.75, 48.5) -> (-110.5, 48.5)
  line L115 (-110.5, 48.5) -> (-110.5, 36.5)
  line L116 (-110.5, -14.5) -> (-105.75, -14.5)
  line L117 (-105.75, -14.5) -> (-105.75, -2.5)
  line L118 (-105.75, -2.5) -> (-110.5, -2.5)
  line L119 (-110.5, -2.5) -> (-110.5, -14.5)
  line L120 (-110.5, 53.5) -> (-105.75, 53.5)
  line L121 (-105.75, 53.5) -> (-105.75, 65.5)
  line L122 (-105.75, 65.5) -> (-110.5, 65.5)
  line L123 (-110.5, 65.5) -> (-110.5, 53.5)
  line L124 (-110.5, 2.5) -> (-105.75, 2.5)
  line L125 (-105.75, 2.5) -> (-105.75, 14.5)
  line L126 (-105.75, 14.5) -> (-110.5, 14.5)
  line L127 (-110.5, 14.5) -> (-110.5, 2.5)
  line L128 (-110.5, 19.5) -> (-105.75, 19.5)
  line L129 (-105.75, 19.5) -> (-105.75, 31.5)
  line L130 (-105.75, 31.5) -> (-110.5, 31.5)
  line L131 (-110.5, 31.5) -> (-110.5, 19.5)
  circle A28 centre (-122.25, -122.25) radius 2.5
  arc A29 (122.25, -129.75) -> (129.75, -122.25) centre (122.25, -122.25) ccw
  line L132 (122.25, -129.75) -> (-122.25, -129.75)
  arc A30 (-129.75, -122.25) -> (-122.25, -129.75) centre (-122.25, -122.25) ccw
  line L133 (-129.75, -122.25) -> (-129.75, 122.25)
  arc A31 (-122.25, 129.75) -> (-129.75, 122.25) centre (-122.25, 122.25) ccw
  line L134 (-122.25, 129.75) -> (122.25, 129.75)
  arc A32 (129.75, 122.25) -> (122.25, 129.75) centre (122.25, 122.25) ccw
  line L135 (129.75, 122.25) -> (129.75, -122.25)
  arc A33 (38.5, 124.5) -> (29.5, 124.5) centre (34, 118.5) ccw
  arc A34 (38.5, 112.5) -> (38.5, 124.5) centre (34, 118.5) ccw
  arc A35 (29.5, 112.5) -> (38.5, 112.5) centre (34, 118.5) ccw
  arc A36 (29.5, 124.5) -> (29.5, 112.5) centre (34, 118.5) ccw
  circle A37 centre (34, 118.5) radius 7.5
  arc A38 (21.5, 124.5) -> (12.5, 124.5) centre (17, 118.5) ccw
  arc A39 (21.5, 112.5) -> (21.5, 124.5) centre (17, 118.5) ccw
  arc A40 (12.5, 112.5) -> (21.5, 112.5) centre (17, 118.5) ccw
  arc A41 (12.5, 124.5) -> (12.5, 112.5) centre (17, 118.5) ccw
  circle A42 centre (17, 118.5) radius 7.5
extrude "Extrude3'''''" add sketch "Sketch4 (3)" along normal blind 0.5 contours A0 L0 L1 L2 L3 L4 A1 A6 L20 L21 L22 L23 L24 A7 A38 A39 A40 A41 A42 | L25 L26 L27 A41 A42 | L0 L1 L2 L3 L4 A40 A42 | L20 L21 L22 L23 L24 A38 A42 | L5 L19 A36 A37 A39 A42 | A2 L6 L7 L8 L9 L10 A3 A4 L14 L15 L16 L17 L18 A5 A33 A34 A35 A36 A37 | L6 L7 L8 L9 L10 A35 A37 | L14 L15 L16 L17 L18 A33 A37 | L11 L12 L13 A34 A37 picked at (20.654701, 118.5) picked at (8.839691, 118.678175) picked at (14.787432, 115.231405) picked at (14.787432, 121.768595) picked at (25.874809, 117.460712) picked at (37.654701, 118.5) picked at (33.960144, 116.531842) picked at (33.960144, 120.468158) picked at (42.166667, 118.5) bodies 47 in component "bolt-holder_3d"
move_face "OffsetFaces1" offset -0.2 10 faces at (-41.166667, -112.5, -16.166667) (-34, -111, -15.166667) (-24.166667, -112.5, -16.333333) (-17, -111, -15.166667) (-9.833333, -112.5, -16.166667) (-41.166667, -124.5, -16.166667) (-34, -126, -15.166667) (-26.833333, -124.5, -17.166667) (-17, -126, -15.166667) (-9.833333, -124.5, -16.166667) on bodies 47 in component "bolt-holder_3d"
mirror "Mirror1'" about plane through (0, 0, 0) normal (1, 0, 0) of bodies 47 makes body 48 in component "bolt-holder_3d"
sketch "Sketch1 (5)" plane through (0, 0, -46) normal (0, 0, -1) x (1, 0, 0) in component "backing_ply"
  arc A0 (-121.529437, 139.207107) -> (-122.236544, 139.5) centre (-122.236544, 138.5) ccw
  line L0 (-122.236544, 139.5) -> (-138.5, 139.5)
  arc A1 (-138.5, 139.5) -> (-139.5, 138.5) centre (-138.5, 138.5) ccw
  line L1 (-139.5, 138.5) -> (-139.5, 122.236544)
  arc A2 (-139.5, 122.236544) -> (-139.207107, 121.529437) centre (-138.5, 122.236544) ccw
  line L2 (-139.207107, 121.529437) -> (-131.088835, 113.411165)
  arc A3 (-131.088835, 113.411165) -> (-113.411165, 131.088835) centre (-122.25, 122.25) ccw
  line L3 (-113.411165, 131.088835) -> (-121.529437, 139.207107) construction
  circle A4 centre (-129.840277, 129.840277) radius 1.6
  line L4 (-137.5, 133.661165) -> (-134.5, 133.661165)
  line L5 (-134.5, 133.661165) -> (-134.5, 127.661165) construction
  line L6 (-134.5, 127.661165) -> (-137.5, 127.661165)
  line L7 (-137.5, 127.661165) -> (-137.5, 133.661165)
  line L8 (-133.661165, 137.5) -> (-127.661165, 137.5)
  line L9 (-127.661165, 137.5) -> (-127.661165, 134.5)
  line L10 (-127.661165, 134.5) -> (-133.661165, 134.5) construction
  line L11 (-133.661165, 134.5) -> (-133.661165, 137.5)
  line L12 (-118.902364, 118.902364) -> (-123.47532, 117.677044)
  line L13 (-123.47532, 117.677044) -> (-126.822956, 121.02468)
  line L14 (-126.822956, 121.02468) -> (-125.597636, 125.597636)
  line L15 (-125.597636, 125.597636) -> (-121.02468, 126.822956)
  line L16 (-121.02468, 126.822956) -> (-117.677044, 123.47532) construction
  line L17 (-117.677044, 123.47532) -> (-118.902364, 118.902364)
  circle A5 centre (122.25, 122.25) radius 2.5 construction
  circle A6 centre (122.25, -122.25) radius 2.5 construction
  circle A7 centre (-122.25, -122.25) radius 2.5 construction
  circle A8 centre (-122.25, 122.25) radius 2.5 construction
  line L18 (-143.5, -143.5) -> (-143.5, 143.5)
  line L19 (-143.5, 143.5) -> (143.5, 143.5)
  line L20 (143.5, 143.5) -> (143.5, -143.5)
  line L21 (143.5, -143.5) -> (-143.5, -143.5)
  arc A9 (121.529437, -139.207107) -> (122.236544, -139.5) centre (122.236544, -138.5) ccw construction
  line L22 (122.236544, -139.5) -> (138.5, -139.5) construction
  arc A10 (138.5, -139.5) -> (139.5, -138.5) centre (138.5, -138.5) ccw construction
  line L23 (139.5, -138.5) -> (139.5, -122.236544) construction
  arc A11 (139.5, -122.236544) -> (139.207107, -121.529437) centre (138.5, -122.236544) ccw construction
  line L24 (139.207107, -121.529437) -> (131.088835, -113.411165) construction
  arc A12 (131.088835, -113.411165) -> (113.411165, -131.088835) centre (122.25, -122.25) ccw construction
  line L25 (113.411165, -131.088835) -> (121.529437, -139.207107) construction
  circle A13 centre (129.840277, -129.840277) radius 1.6
  line L26 (137.5, -133.661165) -> (134.5, -133.661165) construction
  line L27 (134.5, -133.661165) -> (134.5, -127.661165) construction
  line L28 (134.5, -127.661165) -> (137.5, -127.661165) construction
  line L29 (137.5, -127.661165) -> (137.5, -133.661165) construction
  line L30 (133.661165, -137.5) -> (127.661165, -137.5) construction
  line L31 (127.661165, -137.5) -> (127.661165, -134.5) construction
  line L32 (127.661165, -134.5) -> (133.661165, -134.5) construction
  line L33 (133.661165, -134.5) -> (133.661165, -137.5) construction
  line L34 (118.902364, -118.902364) -> (123.47532, -117.677044) construction
  line L35 (123.47532, -117.677044) -> (126.822956, -121.02468) construction
  line L36 (126.822956, -121.02468) -> (125.597636, -125.597636) construction
  line L37 (125.597636, -125.597636) -> (121.02468, -126.822956) construction
  line L38 (121.02468, -126.822956) -> (117.677044, -123.47532) construction
  line L39 (117.677044, -123.47532) -> (118.902364, -118.902364) construction
  arc A14 (-139.207107, -121.529437) -> (-139.5, -122.236544) centre (-138.5, -122.236544) ccw construction
  line L40 (-139.5, -122.236544) -> (-139.5, -138.5) construction
  arc A15 (-139.5, -138.5) -> (-138.5, -139.5) centre (-138.5, -138.5) ccw construction
  line L41 (-138.5, -139.5) -> (-122.236544, -139.5) construction
  arc A16 (-122.236544, -139.5) -> (-121.529437, -139.207107) centre (-122.236544, -138.5) ccw construction
  line L42 (-121.529437, -139.207107) -> (-113.411165, -131.088835) construction
  arc A17 (-113.411165, -131.088835) -> (-131.088835, -113.411165) centre (-122.25, -122.25) ccw construction
  line L43 (-131.088835, -113.411165) -> (-139.207107, -121.529437) construction
  circle A18 centre (-129.840277, -129.840277) radius 1.6
  line L44 (-133.661165, -137.5) -> (-133.661165, -134.5) construction
  line L45 (-133.661165, -134.5) -> (-127.661165, -134.5) construction
  line L46 (-127.661165, -134.5) -> (-127.661165, -137.5) construction
  line L47 (-127.661165, -137.5) -> (-133.661165, -137.5) construction
  line L48 (-137.5, -133.661165) -> (-137.5, -127.661165) construction
  line L49 (-137.5, -127.661165) -> (-134.5, -127.661165) construction
  line L50 (-134.5, -127.661165) -> (-134.5, -133.661165) construction
  line L51 (-134.5, -133.661165) -> (-137.5, -133.661165) construction
  line L52 (-118.902364, -118.902364) -> (-117.677044, -123.47532) construction
  line L53 (-117.677044, -123.47532) -> (-121.02468, -126.822956) construction
  line L54 (-121.02468, -126.822956) -> (-125.597636, -125.597636) construction
  line L55 (-125.597636, -125.597636) -> (-126.822956, -121.02468) construction
  line L56 (-126.822956, -121.02468) -> (-123.47532, -117.677044) construction
  line L57 (-123.47532, -117.677044) -> (-118.902364, -118.902364) construction
  arc A19 (139.207107, 121.529437) -> (139.5, 122.236544) centre (138.5, 122.236544) ccw construction
  line L58 (139.5, 122.236544) -> (139.5, 138.5) construction
  arc A20 (139.5, 138.5) -> (138.5, 139.5) centre (138.5, 138.5) ccw construction
  line L59 (138.5, 139.5) -> (122.236544, 139.5) construction
  arc A21 (122.236544, 139.5) -> (121.529437, 139.207107) centre (122.236544, 138.5) ccw construction
  line L60 (121.529437, 139.207107) -> (113.411165, 131.088835) construction
  arc A22 (113.411165, 131.088835) -> (131.088835, 113.411165) centre (122.25, 122.25) ccw construction
  line L61 (131.088835, 113.411165) -> (139.207107, 121.529437) construction
  circle A23 centre (129.840277, 129.840277) radius 1.6
  line L62 (133.661165, 137.5) -> (133.661165, 134.5) construction
  line L63 (133.661165, 134.5) -> (127.661165, 134.5) construction
  line L64 (127.661165, 134.5) -> (127.661165, 137.5) construction
  line L65 (127.661165, 137.5) -> (133.661165, 137.5) construction
  line L66 (137.5, 133.661165) -> (137.5, 127.661165) construction
  line L67 (137.5, 127.661165) -> (134.5, 127.661165) construction
  line L68 (134.5, 127.661165) -> (134.5, 133.661165) construction
  line L69 (134.5, 133.661165) -> (137.5, 133.661165) construction
  line L70 (118.902364, 118.902364) -> (117.677044, 123.47532) construction
  line L71 (117.677044, 123.47532) -> (121.02468, 126.822956) construction
  line L72 (121.02468, 126.822956) -> (125.597636, 125.597636) construction
  line L73 (125.597636, 125.597636) -> (126.822956, 121.02468) construction
  line L74 (126.822956, 121.02468) -> (123.47532, 117.677044) construction
  line L75 (123.47532, 117.677044) -> (118.902364, 118.902364) construction
extrude "Extrude1''''''" add sketch "Sketch1 (5)" along normal blind 3 separate body makes body 49 in component "backing_ply"